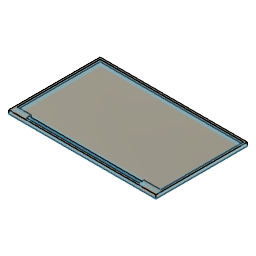
GóraLaptop (Autodesk Fusion 360 design; units mm, degrees)
part number: 2025-11-11-11-04-48-412
Autodesk Fusion 360 part; units mm, degrees
sketch "Szkic1" plane through (0, 0, 0) normal (0, 0, 1) x (1, 0, 0)
  line L0 (-190.7916, 55) -> (169.2084, 55)
  line L1 (169.2084, 55) -> (169.2084, -153)
  line L2 (169.2084, -153) -> (-190.7916, -153)
  line L3 (-190.7916, -153) -> (-190.7916, 55)
  line L4 (-186.2916, 51.8) -> (159.7084, 51.8)
  line L5 (159.7084, 51.8) -> (159.7084, -145.2)
  line L6 (159.7084, -145.2) -> (-186.2916, -145.2)
  line L7 (-186.2916, -145.2) -> (-186.2916, 51.8)
  line L8 (-155.7916, -153) -> (127.2084, -153)
  line L9 (127.2084, -153) -> (127.2084, -164.9)
  line L10 (127.2084, -164.9) -> (-155.7916, -164.9)
  line L11 (-155.7916, -164.9) -> (-155.7916, -153)
  line L12 (-195.7916, 60) -> (174.2084, 60)
  line L13 (174.2084, 60) -> (174.2084, -169.9)
  line L14 (174.2084, -169.9) -> (-195.7916, -169.9)
  line L15 (-195.7916, -169.9) -> (-195.7916, 60)
  dimension "d1" = 360
  dimension "d2" = 208
  dimension "d3" = 346
  dimension "d4" = 197
  dimension "d5" = 9.5
  dimension "d6" = 7.8
  dimension "d7" = 11.9
  dimension "d8" = 35
  dimension "d9" = 283
  dimension "d10" = 370
  dimension "d11" = 5
  dimension "d12" = 5
  dimension "d13" = 5
  constraint horizontal L0
  constraint vertical L1
  constraint horizontal L2
  constraint vertical L3
  constraint horizontal L4
  constraint vertical L5
  constraint horizontal L6
  constraint vertical L7
  constraint horizontal L8
  constraint vertical L9
  constraint horizontal L10
  constraint vertical L11
  constraint coincident L2 L8.start
  constraint horizontal L12
  constraint vertical L13
  constraint horizontal L14
  constraint vertical L15
  measures "d1" distance of L0.start L0.end
  measures "d2" distance of L0.start L2.end
  measures "d3" distance of L4.start L4.end
  measures "d4" distance of L4.start L6.end
  measures "d5" distance of L1 L5
  measures "d6" distance of L2 L6
  measures "d7" distance of L8.start L10.end
  measures "d8" distance of L3 L11
  measures "d9" distance of L9.end L10.end
  measures "d10" distance of L12.start L12.end
  measures "d11" distance of L3 L15
  measures "d12" distance of L10 L14
  measures "d13" distance of L0 L12
extrude "Wyciągnięcie proste1" add sketch "Szkic1" along normal blind 5 contours L12 L13 L14 L15
extrude "Wyciągnięcie proste2" add 1 faces at (156.8751, -162.6, 5) along direction (0, 0, 1) blind 4
extrude "Wyciągnięcie proste3" add sketch "Szkic1" along normal blind 4 contours L0 L1 L2 L3 L8 | L4 L5 L6 L7
